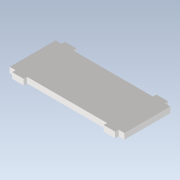
# Autodesk Inventor part: Steckerplatte_seit
Saved by Autodesk Inventor 2022 (Build 260153000, 153)
## iProperties
Created: 2022-02-01
Part Number: Steckerplatte_seit
Material: Generic
Document SubType Name: Modeling
Designer: Fabijansven
Density: 1 g/cm^3
Appearance: Default
Author: Fabijansven
Autodesk Inventor part; units mm, degrees
ref_plane "YZ Plane" through (0, 0, 0) normal (1, 0, 0) x (0, 1, 0)
ref_plane "XZ Plane" through (0, 0, 0) normal (0, 1, 0) x (-1, 0, 0)
ref_plane "XY Plane" through (0, 0, 0) normal (0, 0, 1) x (1, 0, 0)
sketch "Sketch1" plane through (0, 0, 0) normal (0, 1, 0) x (-1, 0, 0)
  line L0 (0, 0) -> (100, 0)
  line L1 (100, 0) -> (100, -40)
  line L2 (100, -40) -> (0, -40)
  line L3 (0, -40) -> (0, 0)
  line L4 (94.9, -40) -> (84.9, -40)
  line L5 (84.9, -40) -> (84.9, -43)
  line L6 (84.9, -43) -> (94.9, -43)
  line L7 (94.9, -43) -> (94.9, -40)
  line L8 (15.1, -40) -> (5.1, -40)
  line L9 (5.1, -40) -> (5.1, -43)
  line L10 (5.1, -43) -> (15.1, -43)
  line L11 (15.1, -43) -> (15.1, -40)
  line L12 (15.1, 0) -> (5.1, 0)
  line L13 (5.1, 0) -> (5.1, 3)
  line L14 (5.1, 3) -> (15.1, 3)
  line L15 (15.1, 3) -> (15.1, 0)
  line L16 (84.9, 0) -> (94.9, 0)
  line L17 (94.9, 0) -> (94.9, 3)
  line L18 (94.9, 3) -> (84.9, 3)
  line L19 (84.9, 3) -> (84.9, 0)
  dimension "d0" = 40
  dimension "d1" = 100
  dimension "d2" = 3
  dimension "d3" = 5.1
  dimension "d4" = 10
  dimension "d5" = 5.1
  dimension "d6" = 10
  dimension "d7" = 5.1
  dimension "d8" = 3
  dimension "d9" = 5.1
  dimension "d10" = 10
  constraints: 40 end point, 10 parallel, 7 point on line, 5 horizontal, 5 perpendicular
  measures "d0" distance of L0.end L1.end
  measures "d1" distance of L1.end L2.end
  measures "d2" distance between parallel lines of L4 L6
  measures "d3" distance between parallel lines of L7 L1
  measures "d4" distance of L5.end L6.end
  measures "d5" distance between parallel lines of L9 L3
  measures "d6" distance of L9.end L10.end
  measures "d7" distance between parallel lines of L3 L13
  measures "d8" distance between parallel lines of L0 L14
  measures "d9" distance between parallel lines of L1 L17
  measures "d10" distance of L17.end L18.end
extrude "Extrusion1" add sketch "Sketch1" along normal blind 5
sketch "Sketch2" plane through (0, 0, 0) normal (0, -1, 0) x (1, 0, 0)
  circle A0 centre (-82, -27.5) radius 9
  line L0 (-100, -40) -> (-100, 0) projected
  line L1 (-15.1, -40) -> (-84.9, -40) projected
  point P0 (0, 0)
  dimension "d13" = 18
  dimension "d14" = 18
  dimension "d15" = 12.5
  constraints: 1 centre point
  measures "d13" diameter of A0
  measures "d14" distance from line of L0 A0.centre
  measures "d15" distance from line of L1 A0.centre
extrude "Extrusion2" cut sketch "Sketch2" against normal blind 5
body "Solid1"
